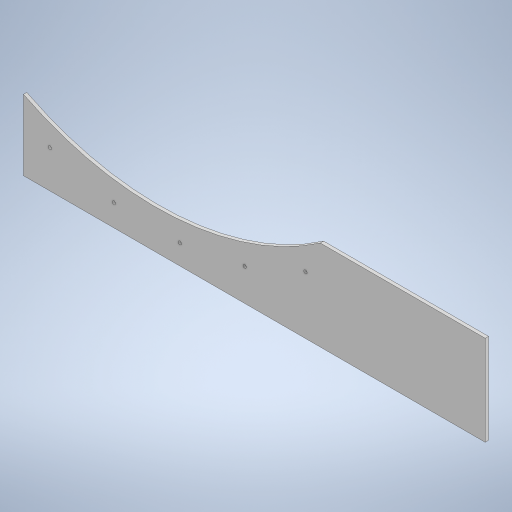
# Autodesk Inventor part: boundaryHalf2V1
Saved by Autodesk Inventor 2024.4 (Build 284460000, 460)
## iProperties
Created: 2025-11-05
Part Number: boundaryHalf2V1
Material: Generic
Document SubType Name: Modeling
Designer: jonas
Density: 1 g/cm^3
Appearance: Default
Author: jonas
Autodesk Inventor part; units mm, degrees
ref_plane "YZ Plane" through (0, 0, 0) normal (1, 0, 0) x (0, 1, 0)
ref_plane "XZ Plane" through (0, 0, 0) normal (0, 1, 0) x (-1, 0, 0)
ref_plane "XY Plane" through (0, 0, 0) normal (0, 0, 1) x (1, 0, 0)
sketch "Sketch2" plane through (0, 0, 0) normal (0, 1, 0) x (-1, 0, 0)
  line L0 (0, 329.241) -> (0, -329.241) construction
  line L1 (203.5937, 0) -> (-203.5937, 0) construction
  arc A0 (-250, -363.4133) -> (200, -393.1529) centre (0, 0) ccw
  line L2 (-500, -363.4133) -> (-500, -500)
  line L3 (-500, -500) -> (200, -500)
  line L4 (200, -500) -> (200, -393.1529)
  line L5 (-250, -363.4133) -> (-500, -363.4133)
  dimension "d0" = 500
  dimension "d2" = 500
  dimension "d3" = 441.1
  dimension "d5" = 363.4133
  dimension "d19" = 700
  constraints: 12 end point, 3 coincident, 3 perpendicular, 2 midpoint, 2 point on circle, 1 centre point, 1 horizontal, 1 vertical
  measures "d0" distance between parallel lines of L2 L0
  measures "d2" distance between parallel lines of L3 L1
  measures "d3" radius of A0
  measures "d5" distance between parallel lines of L1 L5
  measures "d19" distance between parallel lines of L4 L2
extrude "Extrusion1" add sketch "Sketch2" along normal blind 5
sketch "Sketch3" plane through (0, 0, 0) normal (0, -1, 0) x (1, 0, 0)
  line L0 (-160, -443.0973) -> (-62.8707, -466.8859) construction
  line L1 (-62.8707, -466.8859) -> (37.0914, -469.6376) construction
  line L2 (37.0914, -469.6376) -> (135.3823, -451.2282) construction
  line L3 (135.3823, -451.2282) -> (227.5731, -412.4872) construction
  line L4 (-160, -443.0973) -> (0, 0) construction
  line L5 (0, 0) -> (-62.8707, -466.8859) construction
  line L6 (0, 0) -> (37.0914, -469.6376) construction
  line L7 (0, 0) -> (135.3823, -451.2282) construction
  line L8 (0, 0) -> (227.5731, -412.4872) construction
  line L9 (309.5098, -355.1604) -> (227.5731, -412.4872) construction
  line L10 (309.5098, -355.1604) -> (0, 0) construction
  line L11 (-200, -500) -> (-200, -393.1529) construction
  dimension "d8" = 471.1
  dimension "d9" = 100
  dimension "d10" = 40
  constraints: 22 end point, 9 equal length
  measures "d8" distance of L0.start L4.end
  measures "d9" distance of L0.start L0.end
  measures "d10" distance from line of L11 L0.start
hole "Hole1" at (-160, 0, -443.0973) at (-62.8707, 0, -466.8859) at (37.0914, 0, -469.6376) at (135.3823, 0, -451.2282) at (227.5731, 0, -412.4872) at (309.5098, 0, -355.1604) direction (0, 1, 0) diameter 5 end through all
body "Solid1"
